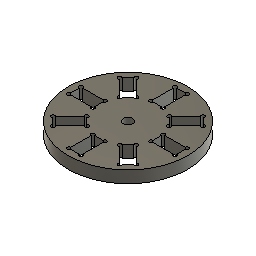
System View (Autodesk Fusion 360 archive; units mm, degrees)
design "Yatsı Mıknatıs Tutucu"
Autodesk Fusion 360 part; units mm, degrees
sketch "Eskiz1" plane through (0, 0, 0) normal (0, 1, 0) x (1, 0, 0)
  circle A0 centre (0, 0) radius 20
  circle A1 centre (0, 0) radius 50
  line L0 (-5, 44.3809) -> (5, 44.3809)
  line L1 (5, 44.3809) -> (5, 24.3809)
  line L2 (5, 24.3809) -> (-5, 24.3809)
  line L3 (-5, 24.3809) -> (-5, 44.3809)
  circle A2 centre (-5, 24.3809) radius 1.5
  circle A3 centre (5, 24.3809) radius 1.5
  circle A4 centre (-5, 44.3809) radius 1.5
  circle A5 centre (5, 44.3809) radius 1.5
  circle A6 centre (-34.9176, 27.8465) radius 1.5
  line L4 (-34.9176, 27.8465) -> (-27.8465, 34.9176)
  line L5 (-20.7754, 13.7044) -> (-34.9176, 27.8465)
  line L6 (-13.7044, 20.7754) -> (-20.7754, 13.7044)
  line L7 (-27.8465, 34.9176) -> (-13.7044, 20.7754)
  circle A7 centre (-27.8465, 34.9176) radius 1.5
  circle A8 centre (-20.7754, 13.7044) radius 1.5
  circle A9 centre (-13.7044, 20.7754) radius 1.5
  circle A10 centre (-44.3809, -5) radius 1.5
  line L8 (-44.3809, -5) -> (-44.3809, 5)
  line L9 (-24.3809, -5) -> (-44.3809, -5)
  line L10 (-24.3809, 5) -> (-24.3809, -5)
  line L11 (-44.3809, 5) -> (-24.3809, 5)
  circle A11 centre (-44.3809, 5) radius 1.5
  circle A12 centre (-24.3809, -5) radius 1.5
  circle A13 centre (-24.3809, 5) radius 1.5
  circle A14 centre (-27.8465, -34.9176) radius 1.5
  line L12 (-27.8465, -34.9176) -> (-34.9176, -27.8465)
  line L13 (-13.7044, -20.7754) -> (-27.8465, -34.9176)
  line L14 (-20.7754, -13.7044) -> (-13.7044, -20.7754)
  line L15 (-34.9176, -27.8465) -> (-20.7754, -13.7044)
  circle A15 centre (-34.9176, -27.8465) radius 1.5
  circle A16 centre (-13.7044, -20.7754) radius 1.5
  circle A17 centre (-20.7754, -13.7044) radius 1.5
  circle A18 centre (5, -44.3809) radius 1.5
  line L16 (5, -44.3809) -> (-5, -44.3809)
  line L17 (5, -24.3809) -> (5, -44.3809)
  line L18 (-5, -24.3809) -> (5, -24.3809)
  line L19 (-5, -44.3809) -> (-5, -24.3809)
  circle A19 centre (-5, -44.3809) radius 1.5
  circle A20 centre (5, -24.3809) radius 1.5
  circle A21 centre (-5, -24.3809) radius 1.5
  circle A22 centre (34.9176, -27.8465) radius 1.5
  line L20 (34.9176, -27.8465) -> (27.8465, -34.9176)
  line L21 (20.7754, -13.7044) -> (34.9176, -27.8465)
  line L22 (13.7044, -20.7754) -> (20.7754, -13.7044)
  line L23 (27.8465, -34.9176) -> (13.7044, -20.7754)
  circle A23 centre (27.8465, -34.9176) radius 1.5
  circle A24 centre (20.7754, -13.7044) radius 1.5
  circle A25 centre (13.7044, -20.7754) radius 1.5
  circle A26 centre (44.3809, 5) radius 1.5
  line L24 (44.3809, 5) -> (44.3809, -5)
  line L25 (24.3809, 5) -> (44.3809, 5)
  line L26 (24.3809, -5) -> (24.3809, 5)
  line L27 (44.3809, -5) -> (24.3809, -5)
  circle A27 centre (44.3809, -5) radius 1.5
  circle A28 centre (24.3809, 5) radius 1.5
  circle A29 centre (24.3809, -5) radius 1.5
  circle A30 centre (27.8465, 34.9176) radius 1.5
  line L28 (27.8465, 34.9176) -> (34.9176, 27.8465)
  line L29 (13.7044, 20.7754) -> (27.8465, 34.9176)
  line L30 (20.7754, 13.7044) -> (13.7044, 20.7754)
  line L31 (34.9176, 27.8465) -> (20.7754, 13.7044)
  circle A31 centre (34.9176, 27.8465) radius 1.5
  circle A32 centre (13.7044, 20.7754) radius 1.5
  circle A33 centre (20.7754, 13.7044) radius 1.5
  circle A34 centre (0, 0) radius 3.9
  point P0 (-5, 0)
  point P1 (5, 0)
  dimension "d1" = 40
  dimension "d2" = 100
  dimension "d3" = 5
  dimension "d4" = 5
  dimension "d5" = 10
  dimension "d6" = 20
  dimension "d9" = 44.3809
  dimension "d10" = 3
  dimension "d11" = 3
  dimension "d12" = 3
  dimension "d13" = 3
  dimension "d15" = 360
  dimension "d16" = 7.8
  constraint coincident A0.centre A1.centre
  constraint concentric A0 A1
  constraint horizontal L0
  constraint vertical L1
  constraint horizontal L2
  constraint vertical L3
  constraint coincident L2.end L3.start
  constraint coincident L1.end L2.start
  constraint coincident L0.start L3.end
  constraint coincident L0.end L1.start
  measures "d1" diameter of A0
  measures "d2" diameter of A1
  measures "d3" distance of A0.centre P0
  measures "d4" distance of A0.centre P1
  measures "d5" distance of L0.start L0.end
  measures "d6" distance of L0.start L2.end
  measures "d9" distance of P0 L0.start
  measures "d10" diameter of A2
  measures "d11" diameter of A3
  measures "d12" diameter of A4
  measures "d13" diameter of A5
  measures "d16" diameter of A34
extrude "Ekstrüde Et1" add sketch "Eskiz1" along normal blind 10 contours A0 | A1
extrude "Ekstrüde Et2" add sketch "Eskiz1" along normal blind 6.5 contours A0
sketch "Eskiz2" plane through (0, 10, 0) normal (0, 1, 0) x (-1, 0, 0)
  arc A0 (-14.765, -21.8361) -> (-14.765, -19.7148) centre (-13.7044, -20.7754) ccw
  line L0 (-14.765, -21.8361) -> (-26.7858, -33.8569)
  arc A1 (-28.9072, -33.8569) -> (-26.7858, -33.8569) centre (-27.8465, -34.9176) ccw
  line L1 (-28.9072, -33.8569) -> (-33.8569, -28.9072)
  arc A2 (-33.8569, -26.7858) -> (-33.8569, -28.9072) centre (-34.9176, -27.8465) ccw
  line L2 (-33.8569, -26.7858) -> (-21.8361, -14.765)
  arc A3 (-19.7148, -14.765) -> (-21.8361, -14.765) centre (-20.7754, -13.7044) ccw
  line L3 (-19.7148, -14.765) -> (-14.765, -19.7148)
  circle A4 centre (0, 0) radius 3.9
  arc A5 (-3.5, -24.3809) -> (-5, -25.8809) centre (-5, -24.3809) ccw
  line L4 (-3.5, -24.3809) -> (3.5, -24.3809)
  arc A6 (5, -25.8809) -> (3.5, -24.3809) centre (5, -24.3809) ccw
  line L5 (5, -25.8809) -> (5, -42.8809)
  arc A7 (3.5, -44.3809) -> (5, -42.8809) centre (5, -44.3809) ccw
  line L6 (3.5, -44.3809) -> (-3.5, -44.3809)
  arc A8 (-5, -42.8809) -> (-3.5, -44.3809) centre (-5, -44.3809) ccw
  line L7 (-5, -42.8809) -> (-5, -25.8809)
  arc A9 (21.8361, -14.765) -> (19.7148, -14.765) centre (20.7754, -13.7044) ccw
  line L8 (21.8361, -14.765) -> (33.8569, -26.7858)
  arc A10 (33.8569, -28.9072) -> (33.8569, -26.7858) centre (34.9176, -27.8465) ccw
  line L9 (33.8569, -28.9072) -> (28.9072, -33.8569)
  arc A11 (26.7858, -33.8569) -> (28.9072, -33.8569) centre (27.8465, -34.9176) ccw
  line L10 (26.7858, -33.8569) -> (14.765, -21.8361)
  arc A12 (14.765, -19.7148) -> (14.765, -21.8361) centre (13.7044, -20.7754) ccw
  line L11 (14.765, -19.7148) -> (19.7148, -14.765)
  arc A13 (25.8809, 5) -> (24.3809, 3.5) centre (24.3809, 5) ccw
  line L12 (25.8809, 5) -> (42.8809, 5)
  arc A14 (44.3809, 3.5) -> (42.8809, 5) centre (44.3809, 5) ccw
  line L13 (44.3809, 3.5) -> (44.3809, -3.5)
  arc A15 (42.8809, -5) -> (44.3809, -3.5) centre (44.3809, -5) ccw
  line L14 (42.8809, -5) -> (25.8809, -5)
  arc A16 (24.3809, -3.5) -> (25.8809, -5) centre (24.3809, -5) ccw
  line L15 (24.3809, -3.5) -> (24.3809, 3.5)
  arc A17 (14.765, 21.8361) -> (14.765, 19.7148) centre (13.7044, 20.7754) ccw
  line L16 (14.765, 21.8361) -> (26.7858, 33.8569)
  arc A18 (28.9072, 33.8569) -> (26.7858, 33.8569) centre (27.8465, 34.9176) ccw
  line L17 (28.9072, 33.8569) -> (33.8569, 28.9072)
  arc A19 (33.8569, 26.7858) -> (33.8569, 28.9072) centre (34.9176, 27.8465) ccw
  line L18 (33.8569, 26.7858) -> (21.8361, 14.765)
  arc A20 (19.7148, 14.765) -> (21.8361, 14.765) centre (20.7754, 13.7044) ccw
  line L19 (19.7148, 14.765) -> (14.765, 19.7148)
  arc A21 (-5, 25.8809) -> (-3.5, 24.3809) centre (-5, 24.3809) ccw
  line L20 (-5, 25.8809) -> (-5, 42.8809)
  arc A22 (-3.5, 44.3809) -> (-5, 42.8809) centre (-5, 44.3809) ccw
  line L21 (-3.5, 44.3809) -> (3.5, 44.3809)
  arc A23 (5, 42.8809) -> (3.5, 44.3809) centre (5, 44.3809) ccw
  line L22 (5, 42.8809) -> (5, 25.8809)
  arc A24 (3.5, 24.3809) -> (5, 25.8809) centre (5, 24.3809) ccw
  line L23 (3.5, 24.3809) -> (-3.5, 24.3809)
  arc A25 (-33.8569, 28.9072) -> (-33.8569, 26.7858) centre (-34.9176, 27.8465) ccw
  line L24 (-33.8569, 28.9072) -> (-28.9072, 33.8569)
  arc A26 (-26.7858, 33.8569) -> (-28.9072, 33.8569) centre (-27.8465, 34.9176) ccw
  line L25 (-26.7858, 33.8569) -> (-14.765, 21.8361)
  arc A27 (-14.765, 19.7148) -> (-14.765, 21.8361) centre (-13.7044, 20.7754) ccw
  line L26 (-14.765, 19.7148) -> (-19.7148, 14.765)
  arc A28 (-21.8361, 14.765) -> (-19.7148, 14.765) centre (-20.7754, 13.7044) ccw
  line L27 (-21.8361, 14.765) -> (-33.8569, 26.7858)
  arc A29 (-44.3809, -3.5) -> (-42.8809, -5) centre (-44.3809, -5) ccw
  line L28 (-44.3809, -3.5) -> (-44.3809, 3.5)
  arc A30 (-42.8809, 5) -> (-44.3809, 3.5) centre (-44.3809, 5) ccw
  line L29 (-42.8809, 5) -> (-25.8809, 5)
  arc A31 (-24.3809, 3.5) -> (-25.8809, 5) centre (-24.3809, 5) ccw
  line L30 (-24.3809, 3.5) -> (-24.3809, -3.5)
  arc A32 (-25.8809, -5) -> (-24.3809, -3.5) centre (-24.3809, -5) ccw
  line L31 (-25.8809, -5) -> (-42.8809, -5)
  circle A33 centre (0, 0) radius 50

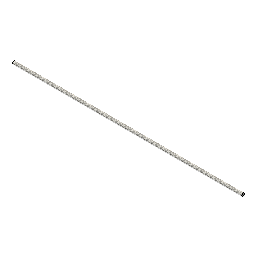
design "Tij Taslak"
Autodesk Fusion 360 part; units mm, degrees
sketch "Eskiz1" plane through (0, 0, 0) normal (1, 0, 0) x (0, 0, -1)
  circle A0 centre (0, 0) radius 4
  dimension "d1" = 8
  constraint coincident A0.centre origin
  measures "d1" diameter of A0
extrude "Ekstrüde Et1" add sketch "Eskiz1" along normal blind 700
thread "Diş1" "ISO Metric profile 8.0 M8x0.8 6g" major diameter 7.901 minor diameter 6.9838 pitch 0.8 angle 60 resizes the face on face at (233.3333, -0.9225, -3.8922)
chamfer "Oluk2" distance 3.9 angle 45 1 faces at (0, 0.7523, -0.0139)

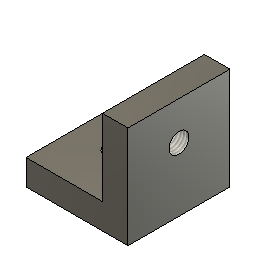
design "Profil Tutucu"
Autodesk Fusion 360 part; units mm, degrees
sketch "Eskiz1" plane through (0, 0, 0) normal (0, 1, 0) x (1, 0, 0)
  circle A0 centre (15, -20) radius 4.5
  line L0 (0, 0) -> (30, 0)
  line L1 (30, 0) -> (30, -40)
  line L2 (30, -40) -> (0, -40)
  line L3 (0, -40) -> (0, 0)
  line L4 (30, 0) -> (40, 0)
  line L5 (40, 0) -> (40, -40)
  line L6 (40, -40) -> (30, -40)
  line L7 (30, -40) -> (30, 0)
  dimension "d3" = 9
  dimension "d13" = 40
  dimension "d25" = 10
  dimension "d31" = 30
  constraint horizontal L0
  constraint vertical L1
  constraint horizontal L2
  constraint vertical L3
  constraint coincident L0.start L3.end
  constraint horizontal L4
  constraint vertical L5
  constraint horizontal L6
  constraint vertical L7
  measures "d3" diameter of A0
  measures "d13" distance of L0.start L2.end
  measures "d25" distance of L0.end L4.end
  measures "d31" distance of L0.start L0.end
extrude "Ekstrüde Et9" add sketch "Eskiz1" along normal blind 10 contours A0 | L0 L1 L2 L3 L7
extrude "Ekstrüde Et10" add sketch "Eskiz1" along normal blind 40 contours L1 L4 L5 L6 L7
sketch "Eskiz4" plane through (30, 0, 0) normal (-1, 0, 0) x (0, 0, 1)
  line L0 (0, 10) -> (40, 10)
  line L1 (40, 10) -> (40, 40)
  line L2 (40, 40) -> (0, 40)
  line L3 (0, 40) -> (0, 10)
  circle A0 centre (20, 25) radius 4.5
  dimension "d36" = 9
  dimension "d37" = 15
  measures "d36" diameter of A0
  measures "d37" distance of L2 A0.centre
hole "Delik1" at (15.0452, 0, 20.1858) direction (0, 1, 0) diameter 7.779 depth 18 tip angle 118
thread "Diş3" "ISO Metric profile 9.0 M9x1.25 6H" major diameter 9.1702 minor diameter 7.7793 pitch 1.25 angle 60 resizes the face on face at (15.2391, 3.3333, 16.3011)
hole "Delik2" at (30, 25, 20) direction (1, 0, 0) diameter 7.779 depth 18 tip angle 118
thread "Diş4" "ISO Metric profile 9.0 M9x1.25 6H"

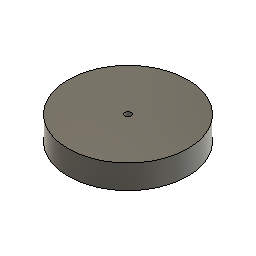
design "Alüminyum Blok Taslak"
Autodesk Fusion 360 part; units mm, degrees
sketch "Eskiz1" plane through (0, 0, 0) normal (0, 1, 0) x (1, 0, 0)
  circle A0 centre (0, 0) radius 75
  circle A1 centre (0, 0) radius 4
  dimension "d1" = 150
  dimension "d2" = 8
  constraint coincident A0.centre A1.centre
  measures "d1" diameter of A0
  measures "d2" diameter of A1
extrude "Ekstrüde Et1" add sketch "Eskiz1" along normal blind 30

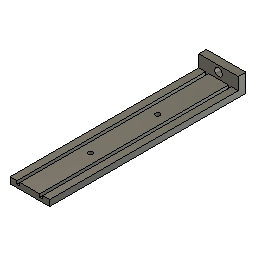
design "İmkansızlar Yan Taraf Kapatıcı"
Autodesk Fusion 360 part; units mm, degrees
sketch "Eskiz1" plane through (0, 0, 0) normal (0, 1, 0) x (1, 0, 0)
  line L0 (0, 0) -> (26, 0)
  line L1 (26, 0) -> (26, -124)
  line L2 (26, -124) -> (0, -124)
  line L3 (0, -124) -> (0, 0)
  line L4 (4.5, 0) -> (6.5, 0)
  line L5 (6.5, 0) -> (6.5, -124)
  line L6 (6.5, -124) -> (4.5, -124)
  line L7 (4.5, -124) -> (4.5, 0)
  line L8 (19.5, 0) -> (21.5, 0)
  line L9 (21.5, 0) -> (21.5, -124)
  line L10 (21.5, -124) -> (19.5, -124)
  line L11 (19.5, -124) -> (19.5, 0)
  line L12 (0, 0) -> (26, 0)
  line L13 (26, 0) -> (26, 5)
  line L14 (26, 5) -> (0, 5)
  line L15 (0, 5) -> (0, 0)
  line L16 (0, -124) -> (26, -124)
  line L17 (26, -124) -> (26, -129)
  line L18 (26, -129) -> (0, -129)
  line L19 (0, -129) -> (0, -124)
  dimension "d1" = 26
  dimension "d2" = 124
  dimension "d3" = 2
  dimension "d4" = 4.5
  dimension "d5" = 2
  dimension "d6" = 13
  dimension "d11" = 5
  dimension "d18" = 5
  constraint horizontal L0
  constraint vertical L1
  constraint horizontal L2
  constraint vertical L3
  constraint coincident L0.start L3.end
  constraint horizontal L4
  constraint vertical L5
  constraint horizontal L6
  constraint vertical L7
  constraint coincident L0 L4.start
  constraint horizontal L8
  constraint vertical L9
  constraint horizontal L10
  constraint vertical L11
  constraint coincident L0 L8.start
  constraint horizontal L12
  constraint vertical L13
  constraint horizontal L14
  constraint vertical L15
  constraint horizontal L16
  constraint vertical L17
  constraint horizontal L18
  constraint vertical L19
  measures "d1" distance of L0.start L0.end
  measures "d2" distance of L0.start L2.end
  measures "d3" distance of L4.start L4.end
  measures "d4" distance of L0.start L4.start
  measures "d5" distance of L8.start L8.end
  measures "d6" distance of L4.end L8.start
  measures "d11" distance of L0.start L14.end
  measures "d18" distance of L2.end L18.end
extrude "Ekstrüde Et1" add sketch "Eskiz1" along normal blind 2 contours L0 L2 L4 L5 L6 L7 L12 L16 | L0 L2 L8 L9 L10 L11 L12 L16 makes body 1 at (6.5, 0.6667, 41.3333) makes body 2 at (21.5, 0.6667, 41.3333)
extrude "Ekstrüde Et2" add sketch "Eskiz1" along normal blind 4 contours L0 L2 L3 L7 L12 L16 | L0 L2 L5 L11 L12 L16 | L0 L1 L2 L9 L12 L16 bodies 1 2
extrude "Ekstrüde Et3" add sketch "Eskiz1" along normal blind 12 contours L0 L4 L8 L12 L13 L14 L15 bodies 1
sketch "Eskiz2" plane through (0, 0, -5) normal (0, 0, -1) x (-1, 0, 0)
  line L0 (-26, 0) -> (0, 0)
  line L1 (0, 0) -> (0, 12)
  line L2 (0, 12) -> (-26, 12)
  line L3 (-26, 12) -> (-26, 0)
  circle A0 centre (-13, 8) radius 2.5
  dimension "d14" = 5
  dimension "d15" = 4
  measures "d14" diameter of A0
  measures "d15" distance of L2 A0.centre
extrude "Ekstrüde Et4" cut sketch "Eskiz2" against normal blind 6 contours A0 bodies 1
sketch "Eskiz3" plane through (0, 4, 0) normal (0, 1, 0) x (-1, 0, 0)
  line L0 (-6.5, 0) -> (-6.5, 124)
  line L1 (-6.5, 124) -> (-19.5, 124)
  line L2 (-19.5, 124) -> (-19.5, 0)
  line L3 (-19.5, 0) -> (-6.5, 0)
  circle A0 centre (-13, 84) radius 1.5
  circle A1 centre (-13, 40) radius 1.5
  dimension "d19" = 3
  dimension "d20" = 3
  dimension "d21" = 40
  dimension "d22" = 40
  measures "d19" diameter of A0
  measures "d20" diameter of A1
  measures "d21" distance of L3 A1.centre
  measures "d22" distance of L1 A0.centre
extrude "Ekstrüde Et5" cut sketch "Eskiz3" against normal blind 15 contours A0 | A1 bodies 1

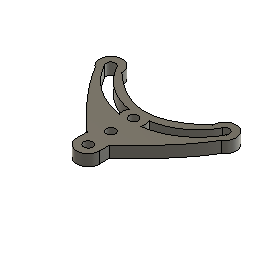
design "İçi Boş Mıknatıs Tutucu"
Autodesk Fusion 360 part; units mm, degrees
sketch "Eskiz2" plane through (0, 0, 0) normal (0, 1, 0) x (1, 0, 0)
  circle A0 centre (0, 0) radius 4
  circle A1 centre (0, 0) radius 10
  circle A2 centre (100, 0) radius 10
  circle A3 centre (100, 0) radius 4
  circle A4 centre (50, -50) radius 10
  circle A5 centre (50, -50) radius 4
  circle A6 centre (50, -70) radius 10
  circle A7 centre (50, -70) radius 4
  circle A8 centre (50, -30) radius 4
  circle A9 centre (50, -30) radius 10
  spline S0 degree 5 poles (0, 10) (2, 7.7246) (6, 3.3724) (12, -2.5597) (20, -9.2571) (30, -15.4718) (40, -19.3367) (50, -20.6598) (60, -19.3367) (70, -15.4718) (80, -9.2571) (88, -2.5597) (94, 3.3724) (98, 7.7246) (100, 10) knots 0 0 0 0 0 0 0.1 0.2 0.3 0.4 0.5 0.6 0.7 0.8 0.9 1 1 1 1 1 1
  arc A10 (50, -26) -> (3.5294, 1.8824) centre (50, 26.6667) ccw
  arc A11 (50, -26) -> (50, -34) centre (50, -30) ccw
  arc A12 (50, -34) -> (-3.5294, -1.8824) centre (50, 26.6667) ccw
  arc A13 (-3.5294, -1.8824) -> (3.5294, 1.8824) centre (0, 0) ccw
  arc A14 (50, -30) -> (0, 0) centre (50, 26.6667) ccw construction
  arc A15 (96.4706, 1.8824) -> (50, -26) centre (50, 26.6667) ccw
  arc A16 (96.4706, 1.8824) -> (103.5294, -1.8824) centre (100, 0) ccw
  arc A17 (103.5294, -1.8824) -> (50, -34) centre (50, 26.6667) ccw
  arc A18 (50, -34) -> (50, -26) centre (50, -30) ccw
  arc A19 (100, 0) -> (50, -30) centre (50, 26.6667) ccw construction
  spline S1 degree 5 poles (-10, 0) (-9.333, -1.3072) (-7.9501, -3.9302) (-5.7286, -7.8903) (-2.4678, -13.2224) (2.1378, -19.9797) (7.3113, -26.8359) (13.0844, -33.7964) (19.4493, -40.8599) (26.3611, -48.0186) (33.7681, -55.2635) (40.0526, -61.1218) (44.9543, -65.5484) (48.3044, -68.5137) (50, -70) knots 0 0 0 0 0 0 0.1 0.2 0.3 0.4 0.5 0.6 0.7 0.8 0.9 1 1 1 1 1 1
  spline S2 degree 5 poles (110, 0) (109.333, -1.3072) (107.9501, -3.9302) (105.7286, -7.8903) (102.4678, -13.2224) (97.8622, -19.9797) (92.6887, -26.8359) (86.9156, -33.7964) (80.5507, -40.8599) (73.6389, -48.0186) (66.2319, -55.2635) (59.9474, -61.1218) (55.0457, -65.5484) (51.6956, -68.5137) (50, -70) knots 0 0 0 0 0 0 0.1 0.2 0.3 0.4 0.5 0.6 0.7 0.8 0.9 1 1 1 1 1 1
  spline S3 degree 5 poles (40.5459, -33.2588) (40.5241, -34.7285) (40.4804, -37.6678) (40.4149, -42.0767) (40.3275, -47.9553) (40.2184, -55.3035) (40.131, -61.1821) (40.0655, -65.5911) (40.0218, -68.5304) (40, -70) knots 0 0 0 0 0 0 0.2 0.4 0.6 0.8 1 1 1 1 1 1
  spline S4 degree 5 poles (60, -70) (59.9782, -68.5304) (59.9345, -65.5911) (59.869, -61.1821) (59.7816, -55.3035) (59.6725, -47.9553) (59.5851, -42.0767) (59.5196, -37.6678) (59.4759, -34.7285) (59.4541, -33.2588) knots 0 0 0 0 0 0 0.2 0.4 0.6 0.8 1 1 1 1 1 1
  point P0 (0, -45)
  point P1 (0, -70)
  point P2 (50, -80)
  point P3 (25, -70)
  point P4 (40, -70)
  point P5 (60, -70)
  point P6 (50, 0)
  point P7 (50, -20)
  point P8 (10, -30)
  point P9 (90, -30)
  point P10 (75, -70)
  point P11 (10, -30)
  point P12 (90, -30)
  dimension "d33" = 8
  dimension "d34" = 20
  dimension "d35" = 8
  dimension "d36" = 20
  dimension "d45" = 100
  dimension "d46" = 8
  dimension "d47" = 20
  dimension "d66" = 8
  dimension "d67" = 20
  dimension "d96" = 8
  dimension "d97" = 20
  dimension "d98" = 20
  dimension "d99" = 30
  dimension "d100" = 40
  dimension "d101" = 40
  dimension "d102" = 8
  dimension "d103" = 8
  dimension "d104" = 25
  constraint coincident A0.centre A1.centre
  constraint concentric A0 A1
  constraint concentric A2 A3
  constraint concentric A4 A5
  constraint concentric A6 A7
  constraint coincident A6 P2
  constraint coincident A6 P4
  constraint coincident A6 P5
  constraint concentric A8 A9
  constraint coincident A1 S0.start
  constraint coincident A9 P7
  constraint coincident A2 S0.end
  constraint tangent A10 A11
  constraint tangent A11 A12
  constraint tangent A12 A13
  constraint tangent A10 A13
  constraint coincident A8.centre A9.centre
  constraint tangent A15 A16
  constraint tangent A16 A17
  constraint tangent A17 A18
  constraint tangent A15 A18
  constraint coincident A2.centre A3.centre
  constraint coincident A1 S1.start
  constraint coincident P11 P8
  constraint coincident A6.centre A7.centre
  constraint coincident A2 S2.start
  constraint coincident P12 P9
  constraint coincident A9 S3.start
  constraint coincident A17 S3.start
  constraint coincident P4 S3.end
  constraint coincident P5 S4.start
  constraint coincident A9 S4.end
  constraint coincident A12 S4.end
  measures "d33" diameter of A0
  measures "d34" diameter of A1
  measures "d35" diameter of A3
  measures "d36" diameter of A2
  measures "d45" distance of A0.centre A2.centre
  measures "d46" diameter of A5
  measures "d47" diameter of A4
  measures "d66" diameter of A7
  measures "d67" diameter of A6
  measures "d96" diameter of A8
  measures "d97" diameter of A9
  measures "d98" distance of A4.centre A8.centre
  measures "d99" distance of A8.centre P6
  measures "d100" distance of A8.centre P11
  measures "d101" distance of A8.centre P12
  measures "d102" diameter of A11
  measures "d103" diameter of A16
  measures "d104" distance of A6.centre P10
extrude "Ekstrüde Et2" add sketch "Eskiz2" along normal blind 10 contours A0 A1 S0 A10 A12 A15 A17 | A1 S0 A10 A15 | A1 A12 A17 S1 | A1 S0 A10 A15 | A1 A9 S0 A15 | A1 A4 A17 S1 S3 | A8 A9 A11 A15 A17 | A9 A10 A15 | A1 S1 | A2 A3 S0 A10 A12 A15 A17 | A2 A12 A17 S2 | A9 A12 A17 | A4 A9 S3 | A2 A9 S0 A10 | A2 S0 A10 A15 | A2 S0 A10 A15 | A8 A9 A10 A12 A18 | A2 S2 | A4 A6 S1 S3 | A6 S1 S3 | A4 A9 S4 | A4 S3 S4 | A4 S3 | A2 S0 A10 A15 | A2 A4 A12 S2 S4 | A6 A7 S1 S2 S3 S4 | A6 A7 S1 S2 | A6 S3 | A4 S4 | A6 S2 S4 | A4 A6 S2 S4 | A6 S4 picked at (7.1423, -1.8575) picked at (6.3904, 6.2)

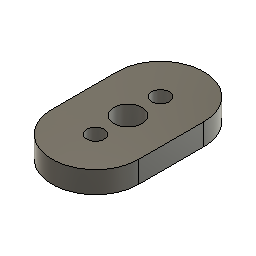
design "Çubuk Tutucu"
Autodesk Fusion 360 part; units mm, degrees
sketch "Eskiz1" plane through (0, 0, 0) normal (0, 1, 0) x (1, 0, 0)
  circle A0 centre (0, 0) radius 6.5
  circle A1 centre (0, 15) radius 4
  circle A2 centre (0, -15) radius 4
  circle A3 centre (0, 15) radius 20
  circle A4 centre (0, -15) radius 20
  line L0 (-20, 15) -> (-20, -15)
  line L1 (20, 15) -> (20, -15)
  dimension "d1" = 13
  dimension "d2" = 8
  dimension "d3" = 8
  dimension "d4" = 15
  dimension "d5" = 15
  dimension "d6" = 40
  dimension "d7" = 40
  constraint coincident A0.centre origin
  constraint concentric A1 A3
  constraint concentric A2 A4
  constraint coincident A3 L0.start
  constraint coincident A4 L0.end
  constraint tangent A4 L0
  constraint vertical L0
  constraint coincident A3 L1.start
  constraint coincident A4 L1.end
  constraint tangent A4 L1
  constraint parallel L0 L1
  measures "d1" diameter of A0
  measures "d2" diameter of A1
  measures "d3" diameter of A2
  measures "d4" distance of A0.centre A1.centre
  measures "d5" distance of A0.centre A2.centre
  measures "d6" diameter of A3
  measures "d7" diameter of A4
extrude "Ekstrüde Et1" add sketch "Eskiz1" along normal blind 10 contours A0 A3 A4 | A0 A3 A4 | A0 A3 A4 | A0 A3 A4 | A3 A4 L1 | A3 A4 L0 picked at (9.7188, 0) picked at (-9.632, 7.9156) picked at (9.632, -7.9156) picked at (-9.7188, 0)
thread "Diş2" [rolled back]

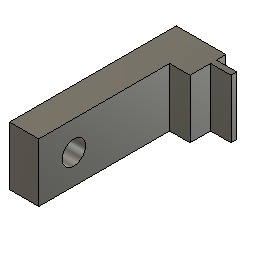
design "İmkansızlar Birleştirme Parçası"
Autodesk Fusion 360 part; units mm, degrees
sketch "Eskiz1" plane through (0, 0, 0) normal (0, 1, 0) x (1, 0, 0)
  line L0 (0, -11.5) -> (0, 0)
  line L1 (0, 0) -> (15, 0)
  line L2 (15, 0) -> (15, -45)
  line L3 (15, -45) -> (0, -45)
  line L4 (0, -45) -> (0, 0)
  dimension "d3" = 15
  dimension "d4" = 45
  constraint vertical L0
  constraint coincident L0.end L1.start
  constraint horizontal L1
  constraint vertical L2
  constraint horizontal L3
  constraint vertical L4
  measures "d3" distance of L0.end L1.end
  measures "d4" distance of L0.end L3.end
extrude "Ekstrüde Et1" add sketch "Eskiz1" along normal blind 20
sketch "Eskiz2" plane through (0, 0, 0) normal (-1, 0, 0) x (0, 0, 1)
  line L0 (0, 0) -> (45, 0)
  line L1 (45, 0) -> (45, 20)
  line L2 (45, 20) -> (0, 20)
  line L3 (0, 20) -> (0, 0)
  line L4 (0, 0) -> (15, 0)
  line L5 (15, 0) -> (15, 20)
  line L6 (15, 20) -> (0, 20)
  line L7 (0, 20) -> (0, 0)
  circle A0 centre (33, 10) radius 4
  point P0 (37, 10)
  dimension "d7" = 15
  dimension "d8" = 20
  dimension "d9" = 8
  dimension "d10" = 8
  constraint horizontal L4
  constraint vertical L5
  constraint horizontal L6
  constraint vertical L7
  constraint coincident L0.start L3.end
  constraint coincident A0 P0
  measures "d7" distance of L0.start L4.end
  measures "d8" distance of L0.start L2.end
  measures "d9" diameter of A0
  measures "d10" distance of L1 P0
extrude "Ekstrüde Et2" cut sketch "Eskiz2" against normal blind 20 contours A0
sketch "Eskiz4" plane through (15, 0, 0) normal (1, 0, 0) x (0, 0, -1)
  circle A0 centre (-33, 10) radius 4
  line L0 (-45, 0) -> (0, 0)
  line L1 (0, 0) -> (0, 20)
  line L2 (0, 20) -> (-45, 20)
  line L3 (-45, 20) -> (-45, 0)
  line L4 (0, 0) -> (-10, 0)
  line L5 (-10, 0) -> (-10, 20)
  line L6 (-10, 20) -> (0, 20)
  line L7 (0, 20) -> (0, 0)
  dimension "d22" = 10
  constraint horizontal L4
  constraint vertical L5
  constraint horizontal L6
  constraint vertical L7
  constraint coincident L0.end L1.start
  measures "d22" distance of L0.end L4.end
extrude "Ekstrüde Et6" add sketch "Eskiz4" along normal blind 7 contours L0 L1 L2 L4 L5 L6 L7
sketch "Eskiz5" plane through (0, 0, 0) normal (0, 0, -1) x (-1, 0, 0)
  line L0 (-22, 0) -> (0, 0)
  line L1 (0, 0) -> (0, 20)
  line L2 (0, 20) -> (-22, 20)
  line L3 (-22, 20) -> (-22, 0)
  line L4 (-22, 0) -> (-15, 0)
  line L5 (-15, 0) -> (-15, 20)
  line L6 (-15, 20) -> (-22, 20)
  line L7 (-22, 20) -> (-22, 0)
  dimension "d25" = 7
  dimension "d26" = 20
  constraint horizontal L4
  constraint vertical L5
  constraint horizontal L6
  constraint vertical L7
  constraint coincident L0.start L3.end
  measures "d25" distance of L0.start L4.end
  measures "d26" distance of L0.start L2.end
extrude "Ekstrüde Et7" add sketch "Eskiz5" along normal blind 12 contours L0 L2 L3 L4 L5 L6 L7
extrude "Ekstrüde Et9" cut 1 faces at (0, 10, 9.6667) along direction (1, 0, 0) blind 5
sketch "Eskiz7" plane through (22, 0, 0) normal (1, 0, 0) x (0, 0, -1)
  line L0 (12, 20) -> (-10, 20)
  line L1 (-10, 20) -> (-10, 0)
  line L2 (-10, 0) -> (12, 0)
  line L3 (12, 0) -> (12, 20)
  line L4 (6.7308, 20) -> (8.7308, 20)
  line L5 (8.7308, 20) -> (8.7308, 0)
  line L6 (8.7308, 0) -> (6.7308, 0)
  line L7 (6.7308, 0) -> (6.7308, 20)
  dimension "d36" = 2
  constraint horizontal L4
  constraint vertical L5
  constraint horizontal L6
  constraint vertical L7
  constraint coincident L0 L4.start
  measures "d36" distance of L4.start L4.end
extrude "Ekstrüde Et10" add sketch "Eskiz7" along normal blind 7 contours L0 L2 L4 L5 L6 L7
extrude "Ekstrüde Et11" add 1 faces at (11.6667, 13.3333, 0) along direction (0, 0, -1) blind 12
extrude "Ekstrüde Et12" cut 1 faces at (17.3333, 6.6667, 10) along direction (0, 0, -1) blind 9.731

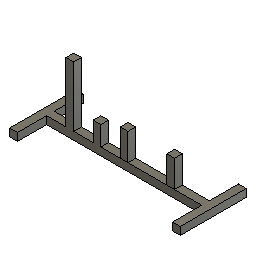
design "Düzenek Taslak"
Autodesk Fusion 360 part; units mm, degrees
sketch "Eskiz1" plane through (0, 0, 0) normal (0, 1, 0) x (1, 0, 0)
  line L0 (0, 0) -> (600, 0)
  line L1 (600, 0) -> (600, -40)
  line L2 (600, -40) -> (0, -40)
  line L3 (0, -40) -> (0, 0)
  line L4 (0, 0) -> (-100, 0)
  line L5 (-100, 0) -> (-100, -40)
  line L6 (-100, -40) -> (0, -40)
  line L7 (0, -40) -> (0, 0)
  line L8 (-100, 0) -> (-140, 0)
  line L9 (-140, 0) -> (-140, -190)
  line L10 (-140, -190) -> (-100, -190)
  line L11 (-100, -190) -> (-100, 0)
  line L12 (-100, -40) -> (-140, -40)
  line L13 (-140, -40) -> (-140, 150)
  line L14 (-140, 150) -> (-100, 150)
  line L15 (-100, 150) -> (-100, -40)
  line L16 (740, 0) -> (740, -190)
  line L17 (700, 0) -> (600, 0)
  line L18 (740, -40) -> (740, 150)
  line L19 (600, -40) -> (700, -40)
  line L20 (700, -190) -> (700, 0)
  line L21 (740, -190) -> (700, -190)
  line L22 (700, -40) -> (700, 0)
  line L23 (740, 150) -> (700, 150)
  line L24 (700, -40) -> (740, -40)
  line L25 (700, 0) -> (740, 0)
  line L26 (700, 150) -> (700, -40)
  dimension "d1" = 600
  dimension "d2" = 40
  dimension "d24" = 100
  dimension "d25" = 40
  dimension "d26" = 40
  dimension "d27" = 190
  dimension "d28" = 40
  dimension "d29" = 190
  dimension "d30" = 100
  dimension "d31" = 40
  dimension "d32" = 40
  dimension "d33" = 190
  dimension "d34" = 40
  dimension "d35" = 190
  constraint horizontal L0
  constraint vertical L1
  constraint horizontal L2
  constraint vertical L3
  constraint coincident L0.start L3.end
  constraint horizontal L4
  constraint vertical L5
  constraint horizontal L6
  constraint vertical L7
  constraint horizontal L8
  constraint vertical L9
  constraint horizontal L10
  constraint vertical L11
  constraint horizontal L12
  constraint vertical L13
  constraint horizontal L14
  constraint vertical L15
  measures "d1" distance of L0.start L0.end
  measures "d2" distance of L0.start L2.end
  measures "d24" distance of L0.start L4.end
  measures "d25" distance of L0.start L2.end
  measures "d26" distance of L4.end L8.end
  measures "d27" distance of L4.end L10.end
  measures "d28" distance of L5.end L12.end
  measures "d29" distance of L5.end L14.end
  measures "d30" distance of L1.end L19.end
  measures "d31" distance of L1.end L0.end
  measures "d32" distance of L18.start L19.end
  measures "d33" distance of L23.end L19.end
  measures "d34" distance of L16.start L17.start
  measures "d35" distance of L20.start L17.start
extrude "Ekstrüde Et1" add sketch "Eskiz1" along normal blind 40 contours L0 L1 L2 L3 L7 makes body 1
sketch "Eskiz2" plane through (0, 40, 0) normal (0, 1, 0) x (-1, 0, 0)
  line L0 (0, 40) -> (-600, 40)
  line L1 (-600, 40) -> (-600, 0)
  line L2 (-600, 0) -> (0, 0)
  line L3 (0, 0) -> (0, 40)
  line L4 (0, 0) -> (-40, 0)
  line L5 (-40, 0) -> (-40, 40)
  line L6 (-40, 40) -> (0, 40)
  line L7 (0, 40) -> (0, 0)
  line L8 (-280, 0) -> (-320, 0)
  line L9 (-320, 0) -> (-320, 40)
  line L10 (-320, 40) -> (-280, 40)
  line L11 (-280, 40) -> (-280, 0)
  line L12 (-520, 0) -> (-560, 0)
  line L13 (-560, 0) -> (-560, 40)
  line L14 (-560, 40) -> (-520, 40)
  line L15 (-520, 40) -> (-520, 0)
  line L16 (-140, 0) -> (-180, 0)
  line L17 (-180, 0) -> (-180, 40)
  line L18 (-180, 40) -> (-140, 40)
  line L19 (-140, 40) -> (-140, 0)
  dimension "d5" = 40
  dimension "d6" = 40
  dimension "d7" = 40
  dimension "d8" = 40
  dimension "d9" = 40
  dimension "d16" = 40
  dimension "d17" = 40
  dimension "d20" = 40
  dimension "d21" = 100
  dimension "d22" = 100
  dimension "d23" = 200
  constraint horizontal L4
  constraint vertical L5
  constraint horizontal L6
  constraint vertical L7
  constraint coincident L2.end L3.start
  constraint horizontal L8
  constraint vertical L9
  constraint horizontal L10
  constraint vertical L11
  constraint coincident L2 L8.start
  constraint horizontal L12
  constraint vertical L13
  constraint horizontal L14
  constraint vertical L15
  constraint coincident L2 L12.start
  constraint horizontal L16
  constraint vertical L17
  constraint horizontal L18
  constraint vertical L19
  constraint coincident L2 L16.start
  measures "d5" distance of L2.end L4.end
  measures "d6" distance of L8.start L8.end
  measures "d7" distance of L8.start L10.end
  measures "d8" distance of L12.start L12.end
  measures "d9" distance of L12.start L14.end
  measures "d16" distance of L16.start L16.end
  measures "d17" distance of L16.start L18.end
  measures "d20" distance of L2.end L0.start
  measures "d21" distance of L4.end L16.start
  measures "d22" distance of L8.start L16.end
  measures "d23" distance of L8.end L12.start
extrude "Ekstrüde Et2" add sketch "Eskiz2" along normal blind 140 separate body contours L0 L2 L8 L9 L10 L11 | L0 L2 L12 L13 L14 L15 makes body 2 at (280, 86.6667, 26.6667) makes body 3 at (520, 86.6667, 26.6667)
extrude "Ekstrüde Et3" add sketch "Eskiz2" along normal blind 310 contours L0 L2 L3 L4 L5 L6 L7 bodies 1
extrude "Ekstrüde Et4" add sketch "Eskiz1" along normal blind 40 contours L3 L4 L5 L6 L7 L11 L15 | L1 L17 L19 L20 L22 L26 | L5 L8 L9 L11 L12 L13 L15 | L8 L13 L14 L15 | L16 L18 L20 L22 L24 L25 L26 | L18 L23 L25 L26 | L9 L10 L11 L12 | L16 L20 L21 L24 bodies 1
extrude "Ekstrüde Et5" add sketch "Eskiz2" along normal blind 100 contours L0 L2 L16 L17 L18 L19 bodies 1

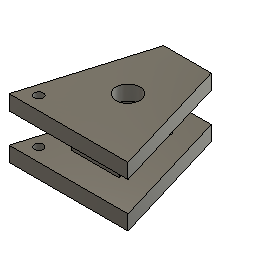
design "Bobin Birleşik"
Autodesk Fusion 360 part; units mm, degrees
sketch "Eskiz1" plane through (0, 0, 0) normal (0, 1, 0) x (1, 0, 0)
  line L0 (0, 0) -> (40, 0)
  line L1 (40, 0) -> (40, -40)
  line L2 (40, -40) -> (0, -40)
  line L3 (0, -40) -> (0, 0)
  line L4 (12, 0) -> (35, 0)
  line L5 (35, -40) -> (12, -40)
  line L6 (12, -40) -> (12, 0)
  line L7 (28, 0) -> (28, -40)
  line L8 (12, 0) -> (0, -40)
  line L9 (28, 0) -> (40, -40)
  circle A0 centre (20, -20) radius 4
  point P0 (12, 0)
  point P1 (28, 0)
  dimension "d1" = 40
  dimension "d2" = 40
  dimension "d3" = 12
  dimension "d4" = 12
  dimension "d5" = 40
  dimension "d23" = 8
  constraint horizontal L0
  constraint vertical L1
  constraint horizontal L2
  constraint vertical L3
  constraint coincident L0.start L3.end
  constraint coincident L0 P0
  constraint coincident L0 P1
  constraint horizontal L4
  constraint horizontal L5
  constraint vertical L6
  constraint coincident L2 L5.start
  constraint coincident P0 L4.start
  constraint vertical L7
  constraint coincident P1 L7.start
  measures "d1" distance of L0.start L0.end
  measures "d2" distance of L0.start L2.end
  measures "d3" distance of L0.start L4.start
  measures "d4" distance of L0.end P1
  measures "d5" distance of P1 L7.end
  measures "d23" diameter of A0
extrude "Ekstrüde Et1" add sketch "Eskiz1" along normal blind 5 contours L0 L2 L4 L5 L6 L7 | L2 L6 L8 | L2 L5 L7 L9 | A0 makes body 1
sketch "Eskiz2" plane through (0, 5, 0) normal (0, 1, 0) x (-1, 0, 0)
  line L0 (-12, 0) -> (0, 40)
  line L1 (0, 40) -> (-40, 40)
  line L2 (-40, 40) -> (-28, 0)
  line L3 (-28, 0) -> (-12, 0)
  line L4 (-12, 0) -> (-28, 0)
  line L5 (-28, 0) -> (-28, 40)
  line L6 (-28, 40) -> (-12, 40)
  line L7 (-12, 40) -> (-12, 0)
  line L8 (-12, 31) -> (-28, 31)
  line L9 (-16, 9) -> (-12, 31)
  line L10 (-24, 9) -> (-28, 31)
  line L11 (-16, 9) -> (-24, 9)
  circle A0 centre (-5.5, 35.5) radius 1.5
  point P0 (-16, 9)
  point P1 (-24, 9)
  point P2 (-12, 35.5)
  point P3 (-5.5, 35.5)
  dimension "d8" = 16
  dimension "d9" = 40
  dimension "d16" = 4
  dimension "d17" = 4
  dimension "d18" = 9
  dimension "d19" = 9
  dimension "d20" = 9
  dimension "d33" = 6.5
  dimension "d34" = 4.5
  dimension "d35" = 3
  constraint horizontal L4
  constraint vertical L5
  constraint horizontal L6
  constraint vertical L7
  constraint coincident L0.start L3.end
  constraint coincident L7 L8.start
  constraint coincident L5 L8.end
  constraint perpendicular L5 L8
  constraint coincident P0 L9.start
  constraint coincident P1 L10.start
  constraint coincident L7 P2
  constraint coincident P3 A0.centre
  measures "d8" distance of L0.start L2.end
  measures "d9" distance of L0.start L6.end
  measures "d16" distance of L7 P0
  measures "d17" distance of L5 P1
  measures "d18" distance of L4 P1
  measures "d19" distance of L4 P0
  measures "d20" distance of L6 L8
  measures "d33" distance of P2 P3
  measures "d34" distance of L8 P2
  measures "d35" diameter of A0
copy_body "CopyPasteBodies1" bodies 1 makes body 2
extrude "Ekstrüde Et4" add sketch "Eskiz2" along normal blind 10 contours L8 L9 L10 L11 bodies 1
move_body "Taşı1" bodies 2 to x (1, 0, 0) y (0, 1, 0) z (0, 0, 1) at (0, 15, 0)
extrude "Ekstrüde Et5" cut sketch "Eskiz1" along normal blind 25 contours A0 bodies 1 2
extrude "Ekstrüde Et6" cut sketch "Eskiz2" along normal blind 19 and the other way blind 8.5 contours A0 bodies 1 2
